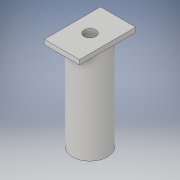
# Autodesk Inventor part: CajonInf
Saved by Autodesk Inventor 2019 (Build 230136000, 136)
## iProperties
Created: 2020-08-08
Part Number: CajonInf
Material: Generic
Document SubType Name: Modeling
Designer: Sergio
Density: 1 g/cm^3
Appearance: Default
Author: Sergio
Autodesk Inventor part; units mm, degrees
ref_plane "YZ Plane" through (0, 0, 0) normal (1, 0, 0) x (0, 1, 0)
ref_plane "XZ Plane" through (0, 0, 0) normal (0, 1, 0) x (-1, 0, 0)
ref_plane "XY Plane" through (0, 0, 0) normal (0, 0, 1) x (1, 0, 0)
sketch "Sketch1" plane through (0, 0, 0) normal (0, 1, 0) x (-1, 0, 0)
  circle A0 centre (0, 0) radius 3.75
  circle A1 centre (0, 0) radius 1.25
  dimension "d0" = 7.5
  dimension "d1" = 2.5
  constraints: 2 centre point, 2 coincident
  measures "d0" diameter of A0
  measures "d1" diameter of A1
extrude "Extrusion1" add sketch "Sketch1" along normal blind 20
sketch "Sketch2" plane through (0, 20, 0) normal (0, 1, 0) x (1, 0, 0)
  line L0 (3.75, 3.75) -> (-3.75, 3.75) construction
  line L1 (-3.75, 3.75) -> (-3.75, -3.75) construction
  line L2 (-3.75, -3.75) -> (3.75, -3.75) construction
  line L3 (3.75, -3.75) -> (3.75, 3.75) construction
  line L4 (3.75, 3.75) -> (-3.75, -3.75) construction
  line L5 (-3.75, 3.75) -> (3.75, -3.75) construction
  line L6 (-3.75, -6) -> (3.75, -6)
  line L7 (3.75, -6) -> (3.75, 6)
  line L8 (3.75, 6) -> (-3.75, 6)
  line L9 (-3.75, 6) -> (-3.75, -6)
  circle A0 centre (0, 0) radius 1.25
  circle A1 centre (0, 0) radius 1.25 projected
  dimension "d4" = 7.5
  dimension "d5" = 7.5
  dimension "d6" = 12
  dimension "d7" = 6
  constraints: 20 end point, 4 parallel, 2 collinear, 2 concentric, 2 horizontal, 2 midpoint, 2 perpendicular, 1 centre point
  measures "d4" distance of L2.end L1.end
  measures "d5" distance of L1.end L0.end
  measures "d6" distance between parallel lines of L8 L6
  measures "d7" distance from line of point (0, 0) L8
extrude "Extrusion2" add sketch "Sketch2" along normal blind 1
body "Solid1"
